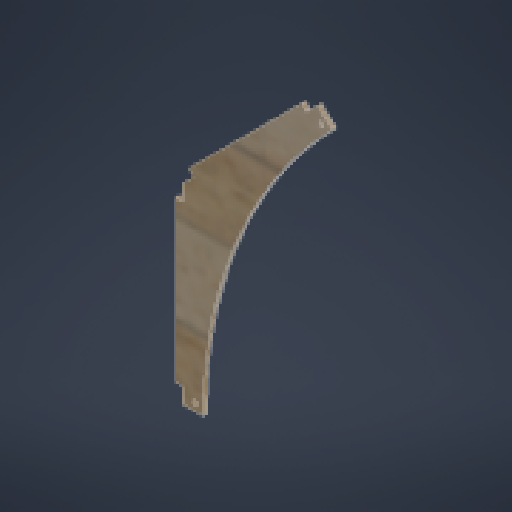
# Autodesk Inventor part: Spcer_curve
Saved by Autodesk Inventor 2026.3 (Build 303398000, 398)
## iProperties
Created: 2026-09-07
Part Number: Spcer_curve
Material: 木材 (カエデ材)
Document SubType Name: Modeling
Designer: takuya
Density: 0.67 g/cm^3
Appearance: ナチュラル カエデ材 - 光沢 濃い着色
Author: takuya
Autodesk Inventor part; units mm, degrees
ref_plane "YZ Plane" through (0, 0, 0) normal (1, 0, 0) x (0, 1, 0)
ref_plane "XZ Plane" through (0, 0, 0) normal (0, 1, 0) x (-1, 0, 0)
ref_plane "XY Plane" through (0, 0, 0) normal (0, 0, 1) x (1, 0, 0)
sketch "スケッチ1" plane through (0, 0, 0) normal (0, 0, 1) x (1, 0, 0)
  line L0 (-5, 0) -> (0, 0) projected
  line L1 (-5, 0) -> (-5, -10) projected
  line L2 (0, -10) -> (-5, -10) projected
  line L3 (0, 0) -> (0, -10) projected
  line L4 (3.5355, 10.6066) -> (7.0711, 7.0711) projected
  line L5 (3.5355, 10.6066) -> (-3.5355, 3.5355) projected
  line L6 (0, 0) -> (-3.5355, 3.5355) projected
  line L7 (7.0711, 7.0711) -> (0, 0) projected
  line L8 (81.6459, 88.717) -> (85.1814, 85.1814) projected
  line L9 (81.6459, 88.717) -> (74.5748, 81.6459) projected
  line L10 (78.1104, 78.1104) -> (74.5748, 81.6459) projected
  line L11 (85.1814, 85.1814) -> (78.1104, 78.1104) projected
  line L12 (-5, -110.4647) -> (0, -110.4647) projected
  line L13 (-5, -110.4647) -> (-5, -120.4647) projected
  line L14 (0, -120.4647) -> (-5, -120.4647) projected
  line L15 (0, -110.4647) -> (0, -120.4647) projected
  line L16 (-4.4431, -120.4647) -> (-4.4431, 1.8404) projected
  line L17 (82.0397, 88.3232) -> (-4.4431, 1.8404) projected
  line L18 (60.4198, 56.1771) -> (5.0711, 0.8284) projected
  line L19 (5.0711, 0.8284) -> (23.6471, -6.866) projected
  arc A0 (60.4198, 56.1771) -> (23.6471, -6.866) centre (290.8276, -120.4647) ccw projected
  line L20 (94.3738, 75.989) -> (87.3027, 83.0601) projected
  arc A1 (87.3027, 83.0601) -> (3, -120.4647) centre (290.8276, -120.4647) ccw projected
  line L21 (13, -120.4647) -> (3, -120.4647) projected
  arc A2 (13.4052, -105.4647) -> (13, -120.4647) centre (290.8276, -120.4647) ccw projected
  arc A3 (94.3738, 75.989) -> (13.4052, -105.4647) centre (290.8276, -120.4647) ccw projected
  line L22 (85.1814, 85.1814) -> (0, 0) projected
  line L23 (0, 0) -> (0, -120.4647) projected
  line L24 (0, -120.4647) -> (3, -120.4647) projected
  arc A4 (87.3027, 83.0601) -> (3, -120.4647) centre (290.8276, -120.4647) ccw projected
  line L25 (87.3027, 83.0601) -> (85.1814, 85.1814) projected
  line L26 (3, -4.1716) -> (21.576, -11.866) projected
  arc A5 (21.576, -11.866) -> (3, -82.4465) centre (290.8276, -120.4647) ccw projected
  line L27 (3, -82.4465) -> (3, -4.1716) projected
  arc A6 (60.4198, 56.1771) -> (23.6471, -6.866) centre (290.8276, -120.4647) ccw projected
  line L28 (23.6471, -6.866) -> (5.0711, 0.8284) projected
  line L29 (5.0711, 0.8284) -> (60.4198, 56.1771) projected
  point P0 (74.9686, 81.2521)
  point P1 (3.9293, 10.2128)
  point P2 (-4.4431, -10)
  point P3 (-4.4431, -110.4647)
  point P4 (-3.1417, 3.1417)
  point P5 (-4.4431, 0)
  point P6 (0, -120.4647)
extrude "押し出し1" add sketch "スケッチ1" against normal blind 2.5 contours L7 L22 L11 L25 A1 L24 L15 L23 L3 | L2 L23 L12 L16 | L4 L17 L10 L22 | A1 L20 A3 A2 L21 | A0 L19 L18 | L26 A5 L27
sketch "スケッチ2" plane through (0, 0, 0) normal (0, 0, 1) x (1, 0, 0)
  circle A0 centre (8.0869, -115.4647) radius 1.5
  circle A1 centre (87.3027, 75.9801) radius 1.5
  point P0 (0, 0)
  constraints: 2 centre point, 4 other
extrude "押し出し2" cut sketch "スケッチ2" against normal blind 10
